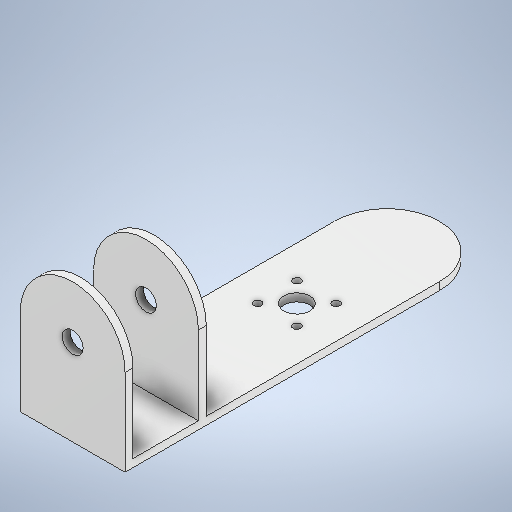
# Autodesk Inventor part: Base_engine
Saved by Autodesk Inventor 2025.3 (Build 293356000, 356)
## iProperties
Created: 2025-07-22
Part Number: Base_engine
Material: Plástico ABS
Document SubType Name: Modeling
Designer: KEVIN
Density: 1.06 g/cm^3
Appearance: Suave - Blanco
Mass: 28.3207 g
Surface Area: 195.823 cm^2
Volume: 26.7177 cm^3
Author: KEVIN
Autodesk Inventor part; units mm, degrees
ref_plane "YZ Plane" through (0, 0, 0) normal (1, 0, 0) x (0, 1, 0)
ref_plane "XZ Plane" through (0, 0, 0) normal (0, 1, 0) x (-1, 0, 0)
ref_plane "XY Plane" through (0, 0, 0) normal (0, 0, 1) x (1, 0, 0)
sketch "Boceto1" plane through (0, 0, 0) normal (1, 0, 0) x (0, 1, 0)
  line L0 (0, 0) -> (0, 60)
  line L1 (0, 0) -> (0, -80)
  line L2 (0, 60) -> (3, 60)
  line L3 (3, -80) -> (0, -80)
  line L4 (3, 60) -> (53, 60)
  line L5 (53, 60) -> (53, 57)
  line L6 (53, 57) -> (3, 57)
  line L7 (3, 32) -> (53, 32)
  line L8 (53, 32) -> (53, 29)
  line L9 (53, 29) -> (3, 29)
  line L10 (3, 57) -> (3, 32)
  line L11 (3, 29) -> (3, -80)
  dimension "d0" = 60
  dimension "d1" = 80
  dimension "d2" = 3
  dimension "d3" = 140
  dimension "d4" = 50
  dimension "d5" = 3
  dimension "d6" = 50
  dimension "d7" = 3
  dimension "d8" = 25
  constraints: 24 end point, 8 perpendicular, 2 horizontal, 2 vertical, 1 parallel
  measures "d0" distance of L0.start L0.end
  measures "d1" distance of L0.start L1.end
  measures "d2" distance of L0.end L2.end
  measures "d3" distance of L2.end L3.start
  measures "d4" distance of L2.end L4.end
  measures "d5" distance of L4.end L5.end
  measures "d6" distance of L7.start L7.end
  measures "d7" distance of L7.end L8.end
  measures "d8" distance between parallel lines of L6 L7
extrude "Extrusión1" add sketch "Boceto1" against normal blind 40
sketch "Boceto2" plane through (0, 3, 29) normal (0, 1, 0) x (1, 0, 0)
  line L0 (-40, 109) -> (-40, -31) projected
  line L1 (0, 109) -> (-40, 109) projected
  arc A0 (0, 89) -> (-40, 89) centre (-20, 89) ccw
  line L2 (0, 89) -> (0, 109)
  line L3 (-40, 109) -> (-40, 89)
  point P0 (0, 29)
  point P1 (-20, 109)
  constraints: 4 end point, 2 point on circle, 1 centre point, 1 parallel, 1 point on line, 1 tangent
extrude "Extrusión2" cut sketch "Boceto2" against normal blind 40
sketch "Boceto3" plane through (0, 0, 60) normal (0, 0, 1) x (1, 0, 0)
  line L0 (0, 53) -> (-40, 53) projected
  arc A0 (0, 33) -> (-40, 33) centre (-20, 33) ccw
  line L1 (-40, 33) -> (-40, 53)
  line L2 (0, 53) -> (0, 33)
  point P0 (0, 0)
  point P1 (-20, 53)
  constraints: 4 end point, 2 point on circle, 1 centre point, 1 tangent, 1 vertical
extrude "Extrusión3" cut sketch "Boceto3" against normal blind 40
sketch "Boceto4" plane through (-40, 0, 60) normal (0, 0, 1) x (1, 0, 0)
  arc A0 (40, 33) -> (0, 33) centre (20, 33) ccw projected
  circle A1 centre (20, 33) radius 4
  point P0 (40, 0)
  dimension "d15" = 8
  constraints: 1 centre point, 1 coincident
  measures "d15" diameter of A1
extrude "Extrusión4" cut sketch "Boceto4" against normal blind 40
sketch "Boceto5" plane through (-40, 3, 29) normal (0, 1, 0) x (1, 0, 0)
  line L0 (0, 0) -> (0, 89.224)
  line L1 (0, 44.612) -> (40, 44.612)
  line L2 (20, 44.612) -> (20, 54.612)
  circle A0 centre (20, 54.612) radius 5
  point P0 (40, 29)
  dimension "d20" = 10
  dimension "d21" = 10
  constraints: 6 end point, 2 midpoint, 2 vertical, 1 centre point, 1 coincident, 1 horizontal
  measures "d20" distance of L2.start L2.end
  measures "d21" diameter of A0
extrude "Extrusión5" cut sketch "Boceto5" against normal blind 40
sketch "Boceto6" plane through (-40, 3, 29) normal (0, 1, 0) x (1, 0, 0)
  line L0 (27.5, 62.112) -> (12.5, 62.112)
  line L1 (12.5, 62.112) -> (12.5, 47.112)
  line L2 (12.5, 47.112) -> (27.5, 47.112)
  line L3 (27.5, 47.112) -> (27.5, 62.112)
  circle A0 centre (20, 54.612) radius 5 projected
  line L4 (27.5, 62.112) -> (12.5, 47.112) construction
  line L5 (12.5, 62.112) -> (27.5, 47.112) construction
  circle A1 centre (12.5, 62.112) radius 1.5
  circle A2 centre (27.5, 62.112) radius 1.5
  circle A3 centre (12.5, 47.112) radius 1.5
  circle A4 centre (27.5, 47.112) radius 1.5
  point P0 (40, 29)
  dimension "d24" = 15
  dimension "d25" = 15
  dimension "d26" = 3
  dimension "d27" = 3
  dimension "d28" = 3
  dimension "d29" = 3
  constraints: 12 end point, 4 centre point, 4 coincident, 2 midpoint, 2 parallel, 1 horizontal, 1 perpendicular
  measures "d24" distance of L2.end L1.end
  measures "d25" distance of L1.end L0.end
  measures "d26" diameter of A1
  measures "d27" diameter of A2
  measures "d28" diameter of A3
  measures "d29" diameter of A4
extrude "Extrusión6" cut sketch "Boceto6" against normal blind 5 contours A1 L1 L0 | L0 L1 A1 | A2 L3 L0 | L0 L3 A2 | A3 L2 L1 | L1 L2 A3 | A4 L2 L3 | L3 L2 A4
